Autodesk Inventor part; units mm, degrees
(part 2 of 2)
extrude "Выдавливание33" cut sketch "Эскиз14" against normal blind 12 from surface at -2 contours L3 L120 A16 L119 A15 L121 A23 L92 L93 L94 L115 L116 L117 L118 | L44 L43 L41 L40 L102 L103 L104 A23 L114 A13 L112 A14 L113 L3 | A23 L104 A12 L114 | L121 A9 L92 A23
extrude "Выдавливание31" cut sketch "Эскиз14" against normal blind 55.6 contours A10 L94 L115 L74 A6 L77 L78 L79 L88 L87 L86 L68 A5 L122 L130 A11 L101 L100 L99 L98 L97 L96 L95 | L130 L122 L60 L40 L102 A11 | L94 L93 L92 A23 L76 L75 L74 L115 | L40 L60 L61 L62 A23 L104 L103 L102 | L115 L26 L122 A5 L68 L86 L87 L88 L79 L78 L77 A6 L74 | L74 L75 L76 A23 L27 L115 | L60 L122 L40 | L40 L29 A23 L62 L61 L60 | L27 A23 L29 L26 | L114 L29 A12 | A12 L104 A23 L62 L114 | L121 L76 A23 L92 A9 | A9 L27 L121 | A23 L76 L27 | L27 A7 L28 L164 A23 | A23 L164 L28 A8 L29 | L29 L62 A23 | L29 A8 L28 A12 | A9 L28 A7 L27 | L28 L80 L81 L82 L164 L108 L107 L106 L105 A12 | L28 L82 L81 L80 | A9 L91 L90 L109 L108 L164 L28 L85 L83 L84 | L84 L83 L85 L28
extrude "Выдавливание34" cut sketch "Эскиз14" against normal blind 25 contours A23 L159 A19 L161 | L161 A2 L159 A23 | L145 A1 L161 A2 | A2 L24 L163 L13 A1 L145 | L24 A3 L162 A0 L13 L163 | A19 L159 L160 L161 | L161 A1 L159 A2 | L145 A22 A1 | A1 L13 L163 A4 L164 L14 L145 A22 L168 L167 L166 | L13 A0 L162 A4 L163 | L159 A1 L145 A2 | A3 L156 A0 L162 | A22 L166 L169 A21 L145 | L145 A21 A22 | L163 L164 A4 | A4 L162 L163 | L145 A1 L14 L164 L23 A2 | L156 L155 L154 A3 L21 L20 L19 | A3 L19 A0 L156 | A0 L156 L157 L154 L14 L164 A4 L162 | A21 L145 | L145 A21 | L166 L167 L168 A22 | A22 L168 L169 L166 | A4 L164 L162 | A3 L21 A0 L19 | L19 L20 L21 A3 | A0 L22 L154 L157 L156 | A21 L169 L168 A22 L145 | L164 L14 A0 L154 A3 L23 | A0 L22 | A3 L154 A0 L21
extrude "Выдавливание35" cut sketch "Эскиз14" against normal blind 4 from surface at -25 contours A22 L166 L169 A21 L145 | L145 A21 A22 | A21 L145 | L145 A21 | L166 L167 L168 A22 | A22 L168 L169 L166 | A21 L169 L168 A22 L145
extrude "Выдавливание36" cut sketch "Эскиз14" against normal blind 5.4 contours L163 L145 A2 L161 A23 | L163 L24 A2 L145 | L161 A2 L159 A23 | A23 L123 L144 L162 | L145 A1 L161 A2 | A2 L24 L163 L13 A1 L145 | L161 A1 L159 A2 | L159 A2 L145 L132 A23 | L144 L123 L29 L28 A12 L105 L106 L107 L108 L164 L23 A3 L154 L155 L156 L162 | A23 L114 A12 L29 L123 | L145 A22 A1 | A1 L13 L163 A4 L164 L14 L145 A22 L168 L167 L166 | L159 A1 L145 A2 | L132 L27 A9 L121 A23 | A3 L156 A0 L162 | A23 L104 A12 L114 | L121 A9 L92 A23 | A22 L166 L169 A21 L145 | L145 A21 A22 | L163 L164 A4 | L145 A1 L14 L164 L23 A2 | A2 L23 L164 L108 L109 L90 L91 A9 L28 L27 L132 L145 | L29 A12 L28 | L156 L155 L154 A3 L21 L20 L19 | A3 L19 A0 L156 | A0 L156 L157 L154 L14 L164 A4 L162 | L114 L29 A12 | A12 L104 A23 L62 L114 | L121 L76 A23 L92 A9 | A9 L27 L121 | A23 L76 L27 | L27 A7 L28 L164 A23 | A21 L145 | L145 A21 | L166 L167 L168 A22 | A22 L168 L169 L166 | A4 L164 L162 | L27 L28 A9 | A23 L164 L28 A8 L29 | L29 L62 A23 | L29 A8 L28 A12 | A3 L21 A0 L19 | L19 L20 L21 A3 | A0 L22 L154 L157 L156 | A9 L28 A7 L27 | A21 L169 L168 A22 L145 | L164 L14 A0 L154 A3 L23 | L28 L80 L81 L82 L164 L108 L107 L106 L105 A12 | A0 L22 | A3 L154 A0 L21 | L28 L82 L81 L80 | A9 L91 L90 L109 L108 L164 L28 L85 L83 L84 | L84 L83 L85 L28
ref_plane "РабПлоскость8" through (-36.9, -3.2175, 44.2) normal (0, 0, -1) x (-1, 0, 0)
sketch "Эскиз18" plane through (-36.9, -3.2175, 44.2) normal (0, 0, -1) x (-1, 0, 0)
  line L0 (41.6, 3.2175) -> (41.6, 13.4175) projected
  line L1 (41.6, 13.4175) -> (41.6, 5.0175)
  line L2 (41.6, 5.0175) -> (20.65, 5.0175) construction
  line L3 (20.65, 5.0175) -> (20.65, -10.3825) construction
  line L4 (15.55, -0.0825) -> (25.75, -0.0825)
  line L5 (25.75, -0.0825) -> (25.75, -5.2825)
  line L6 (25.75, -5.2825) -> (15.55, -5.2825)
  line L7 (15.55, -5.2825) -> (15.55, -0.0825)
  line L8 (15.55, -0.0825) -> (25.75, -5.2825) construction
  line L9 (25.75, -0.0825) -> (15.55, -5.2825) construction
  point P0 (-36.9, 3.2175)
  point P1 (20.65, -2.6825)
  dimension "d339" = 8.4
  dimension "d340" = 20.95
  dimension "d341" = 15.4
  dimension "d342" = 10.2
  dimension "d343" = 5.2
  constraints: 18 end point, 3 midpoint, 2 horizontal, 2 parallel, 2 perpendicular, 1 point on line
  measures "d339" distance of L0.end L1.end
  measures "d340" distance of L1.end L2.end
  measures "d341" distance of L2.end L3.end
  measures "d342" distance of L5.end L6.end
  measures "d343" distance of L4.end L5.end
extrude "Выдавливание37" cut sketch "Эскиз18" against normal blind 2.1 from surface at -15.2
extrude "Выдавливание38" cut sketch "Эскиз18" along normal blind 2.1 from surface at 15.2
sketch "Эскиз19" plane through (-78.5, 10.2, 0) normal (0, 1, 0) x (1, 0, 0)
  line L0 (0, 0) -> (0, -88.4) projected
  line L1 (0, -88.4) -> (157, -88.4) projected
  line L2 (0, 0) -> (157, 0)
  line L3 (157, 0) -> (157, -88.4)
  line L4 (157, -88.4) -> (0, -88.4)
  line L5 (0, -88.4) -> (0, 0)
  line L6 (157, 0) -> (157, -88.4) projected
  line L7 (157, -44.2) -> (0, -44.2) construction
  line L8 (78.5, -88.4) -> (78.5, 0) construction
  line L9 (1.6, -1.6) -> (155.4, -1.6)
  line L10 (155.4, -1.6) -> (155.4, -86.8)
  line L11 (155.4, -86.8) -> (1.6, -86.8)
  line L12 (1.6, -86.8) -> (1.6, -1.6)
  line L13 (1.6, -1.6) -> (155.4, -86.8) construction
  line L14 (155.4, -1.6) -> (1.6, -86.8) construction
  point P0 (78.5, -44.2)
  dimension "d348" = 157
  dimension "d349" = 88.4
  dimension "d350" = 153.8
  dimension "d351" = 85.2
  constraints: 24 end point, 6 midpoint, 4 parallel, 2 horizontal, 2 perpendicular, 1 vertical
  measures "d348" distance of L1.end L4.end
  measures "d349" distance of L2.end L1.end
  measures "d350" distance of L10.end L11.end
  measures "d351" distance of L9.end L10.end
extrude "Выдавливание39" add sketch "Эскиз19" along normal blind 20
sketch "Эскиз20" plane through (0, 0, 0) normal (0, 0, -1) x (-1, 0, 0)
  line L0 (-78.5, 0) -> (-78.5, 30.2) projected
  line L1 (-78.5, 30.2) -> (78.5, 30.2)
  line L2 (78.5, 30.2) -> (78.5, 30.2)
  line L3 (78.5, 30.2) -> (-78.5, 30.2)
  line L4 (-78.5, 30.2) -> (-78.5, 30.2)
  line L5 (0, 30.2) -> (0, 10.2) construction
  line L6 (0, 10.2) -> (-5, 10.2)
  line L7 (-5, 10.2) -> (-28.8351, 30.2)
  line L8 (-76.9, 30.2) -> (76.9, 30.2) projected
  line L9 (-5, 10.2) -> (26.1145, 10.2) construction
  line L10 (0, 10.2) -> (5, 10.2)
  line L11 (5, 10.2) -> (28.8351, 30.2)
  point P0 (0, 0)
  point P1 (-28.8351, 30.2)
  point P2 (-28.8351, 30.2)
  point P3 (28.8351, 30.2)
  point P4 (28.8351, 30.2)
  dimension "d354" = 157
  dimension "d355" = 0
  dimension "d356" = 20
  dimension "d357" = 5
  dimension "d363" = 140
  constraints: 20 end point, 3 equal length, 3 horizontal, 2 symmetric about line, 1 midpoint, 1 perpendicular, 1 point on line, 1 vertical
  measures "d354" distance of L2.end L3.end
  measures "d355" distance of L1.end L2.end
  measures "d356" distance of L5.start L5.end
  measures "d357" distance of L5.end L6.end
  measures "d363" angle of L9 L7
extrude "Выдавливание40" add sketch "Эскиз20" along normal blind 22.5
extrude "Выдавливание41" add sketch "Эскиз20" against normal blind 22.5 from surface at -88.4
extrude "Выдавливание42" cut sketch "Эскиз10" along normal blind 2 from surface at -6 contours L67 L24 L68 L7 | L7 L54 L9 L50 | L9 L69 L26 L66 | L24 L72 L7 L70 | L7 L63 L9 L58 | L71 L9 L73 L26
sketch "Эскиз21" plane through (-46, 10.2, 61.9) normal (0, 0, 1) x (1, 0, 0)
  line L0 (23.1, -33.5956) -> (23.1, -38.7) construction
  line L1 (23.1, -38.7) -> (-0.9, -38.7) construction
  line L2 (-0.9, -38.7) -> (-0.9, -35.2) construction
  line L3 (-0.9, -35.2) -> (23.1, -35.2) construction
  line L4 (23.1, -35.2) -> (23.1, -38.7) construction
  line L5 (-0.9, -35.2) -> (8.1, -35.2)
  line L6 (8.1, -35.2) -> (8.1, -27.2)
  line L7 (8.1, -27.2) -> (-0.9, -27.2)
  line L8 (-0.9, -27.2) -> (-0.9, -35.2)
  point P0 (46, -10.2)
  dimension "d376" = 24
  dimension "d377" = 3.5
  dimension "d378" = 9
  dimension "d379" = 8
  constraints: 16 end point, 4 parallel, 2 horizontal, 2 perpendicular
  measures "d376" distance of L2.end L3.end
  measures "d377" distance of L1.end L2.end
  measures "d378" distance of L7.end L6.end
  measures "d379" distance of L6.end L5.end
extrude "Выдавливание43" cut sketch "Эскиз21" against normal blind 15
sketch "Эскиз22" plane through (-78.5, 10.2, 0) normal (0, 1, 0) x (1, 0, 0)
  line L0 (0, 0) -> (0, -30.0143) construction
  line L1 (0, 0) -> (157, 0) construction
  line L2 (157, 0) -> (157, -88.4) construction
  line L3 (157, -88.4) -> (0, -88.4) construction
  line L4 (0, -88.4) -> (0, 0) construction
  line L5 (139.0073, -45.7852) -> (139.0073, -5.7) construction
  line L6 (128.5, -5) -> (128.5, -22.5) construction
  line L7 (139.0073, -5.7) -> (128.5, -5.7) construction
  line L8 (128.5, -5.7) -> (128.5, -5.9) construction
  line L9 (128.5, -5.9) -> (139.0073, -5.9) construction
  line L10 (139.0073, -5.9) -> (139.0073, -5.7) construction
  line L11 (128.5, -5.9) -> (132.7, -5.9) construction
  line L12 (132.7, -5.9) -> (146.7, -5.9) construction
  line L13 (146.7, -5.9) -> (146.7, -26.7) construction
  line L14 (146.7, -26.7) -> (132.7, -26.7) construction
  line L15 (132.7, -26.7) -> (132.7, -5.9) construction
  line L16 (146.9, -26.9) -> (146.9, -5.7)
  line L17 (146.9, -5.7) -> (132.5, -5.7)
  line L18 (132.5, -5.7) -> (132.5, -26.9)
  line L19 (132.5, -26.9) -> (146.9, -26.9)
  line L20 (132.7, -5.9) -> (135.6, -5.9) construction
  line L21 (135.6, -5.9) -> (135.6, -12.1) construction
  line L22 (135.6, -12.1) -> (132.7, -12.1) construction
  line L23 (132.7, -12.1) -> (132.7, -5.9) construction
  circle A0 centre (135.6, -12.1) radius 1.75
  line L24 (135.6, -12.1) -> (135.6, -21.6) construction
  line L25 (135.6, -12.1) -> (145.1, -12.1) construction
  circle A1 centre (135.6, -21.6) radius 1.75
  line L26 (132.7, -5.9) -> (144.7, -5.9) construction
  line L27 (144.7, -5.9) -> (144.7, -26.7) construction
  line L28 (144.7, -26.7) -> (132.7, -26.7) construction
  line L29 (132.7, -26.7) -> (132.7, -5.9) construction
  line L30 (144.7, -26.7) -> (146.7, -5.9) construction
  line L31 (132.5, -5.7) -> (128.5, -5.7)
  line L32 (128.5, -5.7) -> (128.5, -26.9)
  line L33 (128.5, -26.9) -> (132.5, -26.9)
  line L34 (132.5, -26.9) -> (132.5, -5.7)
  line L35 (146.9, -5.7) -> (160.2, -5.7) construction
  line L36 (160.2, -5.7) -> (160.2, -26.9) construction
  line L37 (160.2, -26.9) -> (146.9, -26.9) construction
  line L38 (146.9, -26.9) -> (146.9, -5.7) construction
  line L39 (157, -5.7) -> (155.4, -5.7) construction
  line L40 (155.4, -5.7) -> (155.4, -26.9) construction
  line L41 (155.4, -26.9) -> (157, -26.9) construction
  line L42 (157, -26.9) -> (157, -5.7)
  line L43 (157, -44.2) -> (0, -44.2) construction
  line L44 (78.5, 0) -> (78.5, -88.4) construction
  line L45 (157, -5.7) -> (146.9, -5.7)
  line L46 (157, -26.9) -> (146.9, -26.9)
  line L47 (146.9, -61.5) -> (146.9, -82.7)
  line L48 (146.9, -82.7) -> (132.5, -82.7)
  line L49 (132.5, -61.5) -> (146.9, -61.5)
  circle A2 centre (135.6, -76.3) radius 1.75
  circle A3 centre (135.6, -66.8) radius 1.75
  line L50 (132.5, -82.7) -> (128.5, -82.7)
  line L51 (128.5, -82.7) -> (128.5, -61.5)
  line L52 (128.5, -61.5) -> (132.5, -61.5)
  line L53 (132.5, -61.5) -> (132.5, -82.7)
  line L54 (157, -61.5) -> (157, -82.7)
  line L55 (157, -82.7) -> (146.9, -82.7)
  line L56 (157, -61.5) -> (146.9, -61.5)
  line L57 (10.1, -26.9) -> (10.1, -5.7)
  line L58 (10.1, -5.7) -> (24.5, -5.7)
  line L59 (24.5, -5.7) -> (24.5, -26.9)
  line L60 (24.5, -26.9) -> (10.1, -26.9)
  circle A4 centre (21.4, -12.1) radius 1.75
  circle A5 centre (21.4, -21.6) radius 1.75
  line L61 (24.5, -5.7) -> (28.5, -5.7)
  line L62 (28.5, -5.7) -> (28.5, -26.9)
  line L63 (28.5, -26.9) -> (24.5, -26.9)
  line L64 (0, -26.9) -> (0, -5.7)
  line L65 (0, -5.7) -> (10.1, -5.7)
  line L66 (0, -26.9) -> (10.1, -26.9)
  line L67 (0, -82.7) -> (10.1, -82.7)
  line L68 (0, -61.5) -> (10.1, -61.5)
  line L69 (0, -61.5) -> (0, -82.7)
  line L70 (10.1, -61.5) -> (10.1, -82.7)
  line L71 (10.1, -82.7) -> (24.5, -82.7)
  line L72 (24.5, -61.5) -> (10.1, -61.5)
  line L73 (24.5, -61.5) -> (24.5, -82.7)
  line L74 (28.5, -61.5) -> (24.5, -61.5)
  line L75 (28.5, -82.7) -> (28.5, -61.5)
  line L76 (24.5, -82.7) -> (28.5, -82.7)
  circle A6 centre (21.4, -76.3) radius 1.75
  circle A7 centre (21.4, -66.8) radius 1.75
  circle A8 centre (135.6, -12.1) radius 2.25
  line L77 (135.6, -9.85) -> (132.5, -9.85)
  line L78 (135.6, -14.35) -> (132.5, -14.35)
  circle A9 centre (135.6, -21.6) radius 2.25
  line L79 (135.6, -19.35) -> (132.5, -19.35)
  line L80 (135.6, -5.9) -> (135.6, -82.7) construction
  line L81 (135.6, -23.85) -> (132.5, -23.85)
  circle A10 centre (135.6, -76.3) radius 2.25
  line L82 (135.6, -78.55) -> (132.5, -78.55)
  line L83 (135.6, -74.05) -> (132.5, -74.05)
  circle A11 centre (135.6, -66.8) radius 2.25
  line L84 (135.6, -69.05) -> (132.5, -69.05)
  line L85 (135.6, -64.55) -> (132.5, -64.55)
  circle A12 centre (21.4, -12.1) radius 2.25
  line L86 (21.4, -9.85) -> (24.5, -9.85)
  line L87 (21.4, -14.35) -> (24.5, -14.35)
  circle A13 centre (21.4, -21.6) radius 2.25
  line L88 (21.4, -19.35) -> (24.5, -19.35)
  line L89 (21.4, -23.85) -> (24.5, -23.85)
  line L90 (21.4, -78.55) -> (24.5, -78.55)
  circle A14 centre (21.4, -76.3) radius 2.25
  line L91 (21.4, -74.05) -> (24.5, -74.05)
  line L92 (21.4, -69.05) -> (24.5, -69.05)
  circle A15 centre (21.4, -66.8) radius 2.25
  line L93 (21.4, -64.55) -> (24.5, -64.55)
  point P0 (24.5, -23.85)
  dimension "d410" = 157
  dimension "d411" = 88.4
  dimension "d421" = 0.2
  dimension "d422" = 4.2
  dimension "d423" = 14
  dimension "d424" = 20.8
  dimension "d425" = 0.2
  dimension "d426" = 2.9
  dimension "d427" = 6.2
  dimension "d428" = 3.5
  dimension "d429" = 9.5
  dimension "d430" = 90
  dimension "d431" = 3.5
  dimension "d432" = 12
  dimension "d433" = 4
  dimension "d434" = 21.2
  dimension "d435" = 13.3
  dimension "d436" = 21.2
  dimension "d437" = 1.6
  dimension "d442" = 0.5
  dimension "d443" = 0.5
  constraints: 182 end point, 66 symmetric about line, 18 parallel, 16 centre point, 16 point on circle, 16 point on line, 14 perpendicular, 11 horizontal, 4 midpoint, 4 tangent, 2 coincident, 1 vertical, 15 other
  measures "d410" distance of L2.end L3.end
  measures "d411" distance of L1.end L2.end
  measures "d421" distance of L8.end L7.end
  measures "d422" distance of L8.end L11.end
  measures "d423" distance of L13.end L14.end
  measures "d424" distance of L12.end L13.end
  measures "d425" distance between parallel lines of L13 L16
  measures "d426" distance of L21.end L22.end
  measures "d427" distance of L20.end L21.end
  measures "d428" diameter of A0
  measures "d429" distance of L24.start L24.end
  measures "d430" angle of L24 L25
  measures "d431" diameter of A1
  measures "d432" distance of L27.end L28.end
  measures "d433" distance of L33.end L32.end
  measures "d434" distance of L32.end L31.end
  measures "d435" distance of L36.end L37.end
  measures "d436" distance of L35.end L36.end
  measures "d437" distance of L41.end L40.end
  measures "d442" radial gap between concentric circles of A0 A8
  measures "d443" radial gap between concentric circles of A1 A9
fillet "Сопряжение4" radius 1 2 edges at (-30.9, -1.25, 23.2) (-30.9, -1.25, 65.2)
sketch "Эскиз24" plane through (78.5, 0, 88.4) normal (1, 0, 0) x (0, 0, -1)
  line L0 (-22.5, 30.2) -> (0, 30.2) projected
  line L1 (0, 30.2) -> (88.4, 30.2) construction
  line L2 (88.4, 30.2) -> (88.4, 0) construction
  line L3 (88.4, 0) -> (0, 0) construction
  line L4 (0, 0) -> (0, 30.2) construction
  line L5 (44.2, 30.2) -> (44.2, 0) construction
  line L6 (44.2, 30.2) -> (44.2, 22.95) construction
  line L7 (41.7, 22.95) -> (46.7, 22.95) construction
  line L8 (41.7, 20.45) -> (46.7, 20.45)
  line L9 (46.7, 25.45) -> (41.7, 25.45)
  arc A0 (41.7, 25.45) -> (41.7, 20.45) centre (41.7, 22.95) ccw
  arc A1 (46.7, 20.45) -> (46.7, 25.45) centre (46.7, 22.95) ccw
  line L10 (44.2, 22.95) -> (88.4, 22.95) construction
  line L11 (88.4, 22.95) -> (73.4, 22.95) construction
  line L12 (70.9, 22.95) -> (75.9, 22.95) construction
  line L13 (70.9, 20.45) -> (75.9, 20.45)
  line L14 (75.9, 25.45) -> (70.9, 25.45)
  arc A2 (70.9, 25.45) -> (70.9, 20.45) centre (70.9, 22.95) ccw
  arc A3 (75.9, 20.45) -> (75.9, 25.45) centre (75.9, 22.95) ccw
  dimension "d452" = 7.25
  dimension "d453" = 2.5
  dimension "d454" = 5
  dimension "d472" = 15
  dimension "d473" = 2.5
  dimension "d474" = 5
  constraints: 32 end point, 8 point on circle, 8 tangent, 4 centre point, 4 midpoint, 4 parallel, 4 point on line, 3 perpendicular, 1 horizontal
  measures "d452" distance of L5.start L6.end
  measures "d453" distance of L6.end L7.end
  measures "d454" diameter of A1
  measures "d472" distance of L10.end L11.end
  measures "d473" distance of L11.end L12.end
  measures "d474" diameter of A3
extrude "Выдавливание50" cut sketch "Эскиз24" against normal blind 1.6 contours A0 L9 A1 L8
sketch "Эскиз25" plane through (-28.8351, 30.2, 110.9) normal (0, 0, 1) x (1, 0, 0)
  line L0 (-49.6649, 0) -> (0, 0) construction
  line L1 (0, 0) -> (57.67, 0) construction
  line L2 (57.67, 0) -> (57.67, -20) construction
  line L3 (57.67, -20) -> (0, -20) construction
  line L4 (0, -20) -> (0, 0) construction
  line L5 (28.835, -20) -> (28.835, 0) construction
  line L6 (28.835, 0) -> (28.835, -7.25) construction
  line L7 (26.585, -7.25) -> (31.085, -7.25) construction
  line L8 (26.585, -9.75) -> (31.085, -9.75)
  line L9 (31.085, -4.75) -> (26.585, -4.75)
  arc A0 (26.585, -4.75) -> (26.585, -9.75) centre (26.585, -7.25) ccw
  arc A1 (31.085, -9.75) -> (31.085, -4.75) centre (31.085, -7.25) ccw
  line L10 (15.335, 0) -> (42.335, 0)
  line L11 (42.335, 0) -> (42.335, -11)
  line L12 (36.3763, -16) -> (21.2938, -16)
  line L13 (15.335, -11) -> (15.335, 0)
  line L14 (57.6701, 0) -> (33.8351, -20) projected
  line L15 (38.6021, -16) -> (42.335, -12.8677)
  line L16 (42.335, -11) -> (36.3763, -16)
  line L17 (15.335, -11) -> (21.2938, -16)
  point P0 (28.8351, -30.2)
  point P1 (42.335, -16)
  point P2 (15.335, -16)
  dimension "d457" = 57.67
  dimension "d458" = 20
  dimension "d459" = 7.25
  dimension "d460" = 2.25
  dimension "d461" = 5
  dimension "d462" = 27
  dimension "d463" = 16
  dimension "d464" = 5
  dimension "d465" = 5.9588
  dimension "d466" = 5
  dimension "d467" = 5.9588
  constraints: 34 end point, 9 point on line, 5 parallel, 4 midpoint, 4 point on circle, 4 tangent, 3 horizontal, 2 centre point, 2 perpendicular
  measures "d457" distance of L2.end L3.end
  measures "d458" distance of L1.end L2.end
  measures "d459" distance of L5.end L6.end
  measures "d460" distance of L6.end L7.end
  measures "d461" diameter of A1
  measures "d462" distance of point (42.335, -16) point (15.335, -16)
  measures "d463" distance of L10.end point (42.335, -16)
  measures "d464" distance of L11.end point (42.335, -16)
  measures "d465" distance of L12.start point (42.335, -16)
  measures "d466" distance of L13.start point (15.335, -16)
  measures "d467" distance of L12.end point (15.335, -16)
extrude "Выдавливание51" cut sketch "Эскиз25" against normal blind 2 contours A0 L9 A1 L8
extrude "Выдавливание52" cut sketch "Эскиз25" against normal blind 7 from surface at -2 contours A0 L9 A1 L8 | L10 L11 L16 L12 L17 L13
mirror "Зеркальное отражение4" about plane through (-36.9, -3.2175, 44.2) normal (0, 0, -1) of "Выдавливание51", "Выдавливание52"
extrude "Выдавливание53" cut sketch "Эскиз24" along normal blind 1.6 from surface at -157 contours A2 L14 A3 L13
ref_plane "РабПлоскость9" through (78.5, 0, 0) normal (0.7071068, 0, -0.7071068) x (0, 1, 0)
sketch "Эскиз26" plane through (78.5, 0, 0) normal (0.7071068, 0, -0.7071068) x (0, 1, 0)
  line L0 (-28.5, -9.5459) -> (0, 0) construction
  line L1 (30.2, -108.753) -> (30.2, 0) construction
  line L2 (0, 0) -> (30.2, 0) construction
  line L3 (30.2, 0) -> (22.95, 0) construction
  line L4 (22.95, 3.5) -> (22.95, -3.5) construction
  line L5 (19.45, 3.5) -> (19.45, -3.5)
  line L6 (26.45, -3.5) -> (26.45, 3.5)
  arc A0 (26.45, 3.5) -> (19.45, 3.5) centre (22.95, 3.5) ccw
  arc A1 (19.45, -3.5) -> (26.45, -3.5) centre (22.95, -3.5) ccw
  point P0 (0, -55.5079)
  dimension "d478" = 7.25
  dimension "d479" = 3.5
  dimension "d480" = 7
  constraints: 12 end point, 4 point on circle, 4 tangent, 2 centre point, 1 horizontal, 1 midpoint, 1 parallel, 1 point on line, 1 vertical
  measures "d478" distance of L1.end L3.end
  measures "d479" distance of L3.end L4.end
  measures "d480" diameter of A1
extrude "Выдавливание54" cut sketch "Эскиз26" against normal blind 10
mirror "Зеркальное отражение5" about plane through (-36.9, -3.2175, 44.2) normal (0, 0, -1) of "Выдавливание54"
